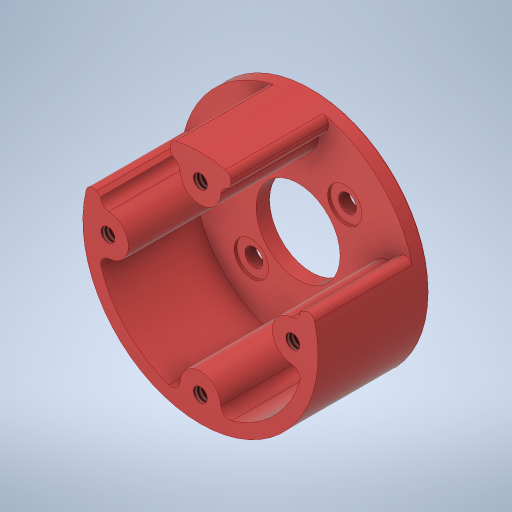
# Autodesk Inventor part: Neo_550_Spacer
Saved by Autodesk Inventor 2023 (Build 270158000, 158)
## iProperties
Created: 2024-01-20
Part Number: Neo_550_Spacer
Material: ABS Plastic
Document SubType Name: Modeling
Designer: mavericks
Density: 1.06 g/cm^3
Appearance: Smooth - Red
Author: mavericks
Autodesk Inventor part; units mm, degrees
ref_plane "YZ Plane" through (0, 0, 0) normal (1, 0, 0) x (0, 1, 0)
ref_plane "XZ Plane" through (0, 0, 0) normal (0, 1, 0) x (-1, 0, 0)
ref_plane "XY Plane" through (0, 0, 0) normal (0, 0, 1) x (1, 0, 0)
sketch "Sketch1" plane through (0, 0, 0) normal (0, 0, 1) x (1, 0, 0)
  circle A0 centre (0, 0) radius 22.225
  dimension "d0" = 44.45
  constraints: 1 centre point, 1 coincident
  measures "d0" diameter of A0
extrude "Extrusion1" add sketch "Sketch1" along normal blind 21
sketch "Sketch2" plane through (0, 0, 21) normal (0, 0, 1) x (1, 0, 0)
  circle A0 centre (0, 0) radius 17.4625 construction
  circle A1 centre (0, 0) radius 22.225 projected
  point P0 (0, 17.4625)
  point P1 (-17.4625, 0)
  point P2 (0, -17.4625)
  point P3 (17.4625, 0)
  dimension "d6" = 360
  dimension "d40" = 4.7625
  constraints: 2 vertical alignment, 1 coincident, 7 other
hole "Hole1" at (0, 17.4625, 21) at (-17.4625, 0, 21) at (0, -17.4625, 21) at (17.4625, 0, 21) direction (0, 0, -1) diameter 2.6416 end through all thread size "6-32 UNC" class "2B" standard "ANSI Unified Screw Threads"
shell "Shell1" thickness 2.54 removed faces 1 at (5.3838, 0.0531, 21)
fillet "Fillet1" radius 1.5875 8 edges at (-19.3996, 3.3397, 11.77) (-19.3996, -3.3397, 11.77) (3.3397, -19.3996, 11.77) (-3.3397, -19.3996, 11.77) (19.3996, -3.3397, 11.77) (19.3996, 3.3397, 11.77) (3.3397, 19.3996, 11.77) (-3.3397, 19.3996, 11.77)
sketch "Sketch3" plane through (0, -17.4625, 2.54) normal (0, 0, 1) x (1, 0, 0)
  circle A0 centre (0, 17.4625) radius 5.715
  line L0 (-5.715, 17.4625) -> (-5.715, 57.8979)
  line L1 (-5.715, 57.8979) -> (5.715, 57.8979)
  line L2 (5.715, 57.8979) -> (5.715, 17.4625)
  line L3 (-3.1339, 12.6834) -> (-43.9105, 39.4226)
  line L4 (-43.9105, 39.4226) -> (43.9105, 39.4226)
  line L5 (43.9105, 39.4226) -> (3.1339, 12.6834)
  arc A1 (-17.3184, 13.6044) -> (-17.3184, 21.3206) centre (-17.4625, 17.4625) ccw projected
  arc A2 (17.3184, 21.3206) -> (17.3184, 13.6044) centre (17.4625, 17.4625) ccw projected
  point P0 (5.715, 39.4226)
  point P1 (-5.715, 39.4226)
  dimension "d17" = 11.43
  constraints: 12 end point, 5 tangent, 4 point on circle, 2 perpendicular, 1 centre point, 1 coincident, 1 parallel, 1 vertical
  measures "d17" diameter of A0
extrude "Extrusion2" cut sketch "Sketch3" along normal blind 20 contours L2 L4 L5 A0 | A0 L3 L4 L0
fillet "Fillet2" radius 1.27 6 edges at (-21.0944, 6.9985, 11.77) (-5.715, 21.4776, 11.77) (-5.715, 18.8234, 11.787) (5.715, 21.4776, 11.77) (5.715, 18.8234, 11.7671) (21.0944, 6.9985, 11.77)
sketch "Sketch4" plane through (0, 17.4625, 2.54) normal (0, 0, 1) x (1, 0, 0)
  circle A0 centre (0, -17.4625) radius 7.9375
  dimension "d21" = 15.875
  constraints: 1 centre point, 1 coincident
  measures "d21" diameter of A0
extrude "Extrusion3" cut sketch "Sketch4" against normal through all
chamfer "Chamfer1" distance 0.2 angle 45 1 edges at (-22.225, 0, 0)
sketch "Sketch5" plane through (0, 17.4625, 2.54) normal (0, 0, 1) x (1, 0, 0)
  circle A0 centre (0, -17.4625) radius 12.5 construction
  circle A1 centre (0, -0.1284) radius 1.4422 construction
  line L0 (-8.8388, -8.6237) -> (0, -17.4625) construction
  line L1 (0, -17.4625) -> (0, -0.1284) construction
  point P0 (-8.8388, -26.3013)
  point P1 (8.8388, -26.3013)
  point P2 (8.8388, -8.6237)
  dimension "d39" = 25
  dimension "d27" = 45
  dimension "d30" = 360
  constraints: 4 end point, 1 centre point, 1 coincident, 1 vertical, 8 other
  measures "d27" angle of L0 L1
hole "Hole2" at (-8.8388, 8.8388, 2.54) at (-8.8388, -8.8388, 2.54) at (8.8388, -8.8388, 2.54) at (8.8388, 8.8388, 2.54) direction (0, 0, -1) diameter 3.4036 end through all counterbore diameter 6.5024 counterbore depth 0.5 clearance for "Socket Head Cap Screw" size "M3" standard "Ansi Metric M Profile"
body "Solid1"
